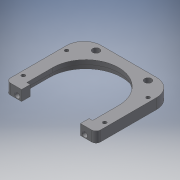
# Autodesk Inventor part: frame top
Saved by Autodesk Inventor 2017 (Build 210142000, 142)
## iProperties
Created: 2018-01-19
Part Number: frame top
Material: Generic
Document SubType Name: Modeling
Designer: RLanting
Density: 1 g/cm^3
Appearance: Default
Author: RLanting
Autodesk Inventor part; units mm, degrees
ref_plane "YZ Plane" through (0, 0, 0) normal (1, 0, 0) x (0, 1, 0)
ref_plane "XZ Plane" through (0, 0, 0) normal (0, 1, 0) x (-1, 0, 0)
ref_plane "XY Plane" through (0, 0, 0) normal (0, 0, 1) x (1, 0, 0)
sketch "Sketch1" plane through (0, 0, 0) normal (0, 0, 1) x (1, 0, 0)
  circle A0 centre (0, 0) radius 4
  circle A1 centre (0, 0) radius 40 construction
  circle A2 centre (0, 0) radius 42 construction
  arc A3 (42, 0) -> (-42, 0) centre (0, 0) ccw
  line L0 (-42, 0) -> (-52, 0)
  line L1 (-52, 0) -> (-52, 50)
  line L2 (-52, 50) -> (52, 50)
  line L3 (52, 50) -> (52, 0)
  line L4 (52, 0) -> (42, 0)
  line L5 (-52, 0) -> (-42, 0)
  line L6 (-42, 0) -> (-42, -40)
  line L7 (-42, -40) -> (-52, -40)
  line L8 (-52, -40) -> (-52, 0)
  line L9 (52, 0) -> (42, 0)
  line L10 (42, 0) -> (42, -40)
  line L11 (42, -40) -> (52, -40)
  line L12 (52, -40) -> (52, 0)
  dimension "d0" = 8
  dimension "d1" = 80
  dimension "d2" = 2
  dimension "d3" = 50
  dimension "d4" = 10
  dimension "d5" = 40
  constraints: 26 end point, 8 equal length, 6 perpendicular, 4 coincident, 3 centre point, 3 horizontal alignment, 2 point on circle, 1 horizontal, 1 point on line, 3 other
  measures "d0" diameter of A0
  measures "d1" diameter of A1
  measures "d3" distance of L2.end L3.end
  measures "d4" distance of L3.end L4.end
  measures "d5" distance of L7.end L0.end
extrude "Extrusion1" add sketch "Sketch1" along normal mid plane 7 contours A3 L0 L1 L2 L3 L4 | L4 L12 L11 L10 | L6 L7 L8 L0
sketch "Sketch2" plane through (0, 0, 3.5) normal (0, 0, 1) x (1, 0, 0)
  line L0 (42, 0) -> (42, -40) projected
  line L1 (42, -40) -> (52, -40) projected
  line L2 (52, -40) -> (52, 50) projected
  line L3 (52, 50) -> (-52, 50) projected
  line L4 (-52, 50) -> (-52, -40) projected
  line L5 (-52, -40) -> (-42, -40) projected
  line L6 (-42, -40) -> (-42, 0) projected
  arc A0 (42, 0) -> (-42, 0) centre (0, 0) ccw projected
  arc A1 (38, 0) -> (-38, 0) centre (0, 0) ccw
  line L7 (-38, 0) -> (-38, -40)
  line L8 (-38, -40) -> (-42, -40)
  line L9 (38, 0) -> (38, -40)
  line L10 (42, -40) -> (52, -40) projected
  line L11 (38, -40) -> (42, -40)
  dimension "d11" = 76
  constraints: 8 end point, 3 perpendicular, 2 point on circle, 2 tangent, 1 centre point, 1 coincident, 1 point on line, 1 vertical
  measures "d11" diameter of A1
extrude "Extrusion2" add sketch "Sketch2" along normal blind 5
sketch "Sketch3" plane through (0, 0, 8.5) normal (0, 0, 1) x (1, 0, 0)
  line L0 (47, -25) -> (-47, -25) construction
  line L1 (-47, -25) -> (-47, 25) construction
  line L2 (-47, 25) -> (47, 25) construction
  line L3 (47, 25) -> (47, -25) construction
  line L4 (47, -25) -> (-47, 25) construction
  line L5 (-47, -25) -> (47, 25) construction
  arc A0 (42, 0) -> (-42, 0) centre (0, 0) ccw construction
  line L6 (-42, -40) -> (-42, 0) construction
  line L7 (42, 0) -> (42, -40) construction
  circle A1 centre (-47, 25) radius 2
  circle A2 centre (-47, -25) radius 2
  circle A3 centre (47, -25) radius 2
  circle A4 centre (47, 25) radius 2
  dimension "d12" = 4
  dimension "d13" = 5
  dimension "d14" = 50
  constraints: 12 end point, 4 centre point, 4 coincident, 3 equal radius, 2 midpoint, 2 parallel, 1 horizontal, 1 perpendicular
  measures "d12" diameter of A1
  measures "d13" distance between parallel lines of L6 L1
  measures "d14" distance of L0.end L1.end
extrude "Extrusion3" cut sketch "Sketch3" against normal through all
sketch "Sketch4" plane through (0, 0, 8.5) normal (0, 0, 1) x (1, 0, 0)
  circle A0 centre (-30, 42) radius 4 projected
  circle A1 centre (30, 42) radius 4 projected
  point P0 (0, 0)
extrude "Extrusion4" cut sketch "Sketch4" against normal through all
sketch "Sketch5" plane through (42, -40, -3.5) normal (0, -1, 0) x (1, 0, 0)
  line L0 (10, 0) -> (10, 12) construction
  line L1 (-4, 12) -> (10, 12) construction
  line L2 (-4, 7) -> (-4, 12) projected
  line L3 (-4, 7) -> (0, 7) projected
  line L4 (0, 0) -> (0, 7) projected
  line L5 (10, 0) -> (0, 0) construction
  line L6 (0, 0) -> (0, 7) construction
  line L7 (0, 3.5) -> (-3, 3.5) construction
  circle A0 centre (-3, 3.5) radius 3
  line L8 (-4, 12) -> (-8, 12)
  line L9 (-80, 12) -> (-4, 12) projected
  line L10 (-8, 12) -> (-8, 0)
  line L11 (-8, 0) -> (0, 0)
  point P0 (-42, 3.5)
  dimension "d19" = 6
  dimension "d20" = 4
  constraints: 8 end point, 1 centre point, 1 coincident, 1 horizontal, 1 midpoint, 1 perpendicular, 1 point on line, 1 tangent, 1 vertical
  measures "d19" diameter of A0
  measures "d20" distance of L1.start L8.end
extrude "Extrusion5" add sketch "Sketch5" against normal blind 10
mirror "Mirror1" about plane through (0, 0, 0) normal (1, 0, 0) of "Extrusion5"
fillet "Fillet1" radius 20 2 edges at (52, 50, 2.5) (-52, 50, 2.5)
fillet "Fillet2" radius 5 2 edges at (52, -40, 2.5) (-52, -40, 2.5)
body "Solid1"
